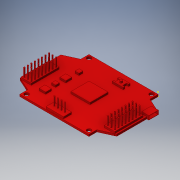
# Autodesk Inventor part: control board
Saved by Autodesk Inventor 2016 (Build 200138000, 138)
## iProperties
Created: 2015-05-25
Part Number: control board
Material: Generic
Document SubType Name: Modeling
Designer: Admin
Density: 1 g/cm^3
Appearance: Default
Mass: 5.47017 g
Surface Area: 80.281 cm^2
Volume: 5.47017 cm^3
Author: Admin
Autodesk Inventor part; units mm, degrees
ref_plane "YZ Plane" through (0, 0, 0) normal (1, 0, 0) x (0, 1, 0)
ref_plane "XZ Plane" through (0, 0, 0) normal (0, 1, 0) x (-1, 0, 0)
ref_plane "XY Plane" through (0, 0, 0) normal (0, 0, 1) x (1, 0, 0)
sketch "Sketch1" plane through (0, 0, 0) normal (0, 1, 0) x (-1, 0, 0)
  circle A0 centre (2.3047, 47.3782) radius 1.524
  line L0 (-0.1112, 0.0907) -> (-0.1112, 49.8747)
  line L1 (-0.1112, 49.8747) -> (-0.1112, 44.1597)
  line L2 (-0.1112, 44.1597) -> (-9.996, 39.6997)
  line L3 (-9.996, 10.5342) -> (-0.1112, 6.0187)
  circle A1 centre (47.3135, 47.3513) radius 1.524
  line L4 (49.6728, 0.0907) -> (49.7323, 49.845)
  line L5 (49.7323, 49.845) -> (49.7255, 44.1597)
  line L6 (49.7255, 44.1597) -> (59.6049, 39.6878)
  line L7 (59.6049, 39.6878) -> (59.5701, 10.5224)
  line L8 (59.5701, 10.5224) -> (49.6799, 6.0187)
  circle A2 centre (21.0522, 45.994) radius 0.4445
  circle A3 centre (23.6023, 45.9907) radius 0.4445
  circle A4 centre (26.1324, 46.0137) radius 0.4445
  circle A5 centre (28.6839, 46.0031) radius 0.4445
  line L9 (-1.4472, 40.2524) -> (-9.0679, 40.2524)
  line L10 (-9.0679, 40.2524) -> (-9.0679, 19.9143)
  line L11 (-9.0679, 19.9143) -> (-1.4472, 19.9143)
  line L12 (-1.4472, 19.9143) -> (-1.4472, 40.2524)
  line L13 (51.1741, 40.1712) -> (58.7055, 40.1712)
  line L14 (58.7055, 40.1712) -> (58.7055, 20.0074)
  line L15 (58.7055, 20.0074) -> (51.1741, 20.0074)
  line L16 (51.1741, 20.0074) -> (51.1741, 40.1712)
  line L17 (18.5986, 43.6399) -> (31.2098, 43.6399)
  line L18 (31.2098, 43.6399) -> (31.2098, 49.4826)
  line L19 (31.2098, 49.4826) -> (18.5986, 49.4901)
  line L20 (18.5986, 49.4901) -> (18.5986, 43.6399)
  line L21 (17.9249, 31.092) -> (31.6611, 31.092)
  line L22 (31.6611, 31.092) -> (31.6611, 18.0268)
  line L23 (31.6611, 18.0268) -> (17.9249, 18.0268)
  line L24 (17.9249, 18.0268) -> (17.9249, 31.092)
  circle A6 centre (-5.2821, 38.9142) radius 0.4445
  circle A7 centre (-2.7297, 38.9142) radius 0.4445
  circle A8 centre (-7.7994, 38.9142) radius 0.4445
  circle A9 centre (-5.2821, 36.3742) radius 0.4445
  circle A10 centre (-2.7297, 36.3742) radius 0.4445
  circle A11 centre (-7.7994, 36.3742) radius 0.4445
  circle A12 centre (-5.2821, 33.8342) radius 0.4445
  circle A13 centre (-2.7297, 33.8342) radius 0.4445
  circle A14 centre (-7.7994, 33.8342) radius 0.4445
  circle A15 centre (-5.2821, 31.2942) radius 0.4445
  circle A16 centre (-2.7297, 31.2942) radius 0.4445
  circle A17 centre (-7.7994, 31.2942) radius 0.4445
  circle A18 centre (-5.2821, 21.1342) radius 0.4445
  circle A19 centre (-2.7297, 21.1342) radius 0.4445
  circle A20 centre (-7.7994, 21.1342) radius 0.4445
  circle A21 centre (-5.2821, 23.6742) radius 0.4445
  circle A22 centre (-2.7297, 23.6742) radius 0.4445
  circle A23 centre (-7.7994, 23.6742) radius 0.4445
  circle A24 centre (-5.2821, 26.2142) radius 0.4445
  circle A25 centre (-2.7297, 26.2142) radius 0.4445
  circle A26 centre (-7.7994, 26.2142) radius 0.4445
  circle A27 centre (-5.2821, 28.7542) radius 0.4445
  circle A28 centre (-2.7297, 28.7542) radius 0.4445
  circle A29 centre (-7.7994, 28.7542) radius 0.4445
  circle A30 centre (54.8719, 38.9142) radius 0.4445
  circle A31 centre (52.3196, 38.9142) radius 0.4445
  circle A32 centre (57.3893, 38.9142) radius 0.4445
  circle A33 centre (54.8719, 36.3742) radius 0.4445
  circle A34 centre (52.3196, 36.3742) radius 0.4445
  circle A35 centre (57.3893, 36.3742) radius 0.4445
  circle A36 centre (54.8719, 33.8342) radius 0.4445
  circle A37 centre (52.3196, 33.8342) radius 0.4445
  circle A38 centre (57.3893, 33.8342) radius 0.4445
  circle A39 centre (54.8719, 31.2942) radius 0.4445
  circle A40 centre (52.3196, 31.2942) radius 0.4445
  circle A41 centre (57.3893, 31.2942) radius 0.4445
  circle A42 centre (54.8719, 21.1342) radius 0.4445
  circle A43 centre (52.3196, 21.1342) radius 0.4445
  circle A44 centre (57.3893, 21.1342) radius 0.4445
  circle A45 centre (54.8719, 23.6742) radius 0.4445
  circle A46 centre (52.3196, 23.6742) radius 0.4445
  circle A47 centre (57.3893, 23.6742) radius 0.4445
  circle A48 centre (54.8719, 26.2142) radius 0.4445
  circle A49 centre (52.3196, 26.2142) radius 0.4445
  circle A50 centre (57.3893, 26.2142) radius 0.4445
  circle A51 centre (54.8719, 28.7542) radius 0.4445
  circle A52 centre (52.3196, 28.7542) radius 0.4445
  circle A53 centre (57.3893, 28.7542) radius 0.4445
  line L25 (15.3968, 9.7927) -> (23.2335, 9.7927)
  line L26 (23.2335, 9.7927) -> (23.2335, 8.6499)
  line L27 (23.2335, 8.6499) -> (21.8717, 8.6499)
  line L28 (21.8717, 8.6499) -> (21.8717, 5.9895)
  line L29 (21.8717, 5.9895) -> (23.2215, 5.9895)
  line L30 (23.2215, 5.9895) -> (23.2215, 4.7481)
  line L31 (23.2215, 4.7481) -> (15.3804, 4.7481)
  line L32 (15.3804, 4.7481) -> (15.3804, 5.8201)
  line L33 (15.3804, 5.8201) -> (16.855, 5.8201)
  line L34 (16.855, 5.8201) -> (16.855, 8.6339)
  line L35 (16.855, 8.6339) -> (15.3133, 8.6339)
  line L36 (15.3133, 8.6339) -> (15.3133, 9.7894)
  line L37 (15.3968, 9.7927) -> (15.3133, 9.7927)
  line L38 (15.3133, 9.7894) -> (15.3133, 9.7927)
  circle A54 centre (19.4197, 7.2385) radius 0.9144
  line L39 (40.3965, 40.5916) -> (45.1465, 40.5916)
  line L40 (45.1465, 40.5916) -> (45.1465, 36.3389)
  line L41 (45.1465, 36.3389) -> (40.3965, 36.3389)
  line L42 (40.3965, 36.3389) -> (40.3965, 40.5916)
  line L43 (41.1619, 32.6713) -> (44.0659, 32.6713)
  line L44 (44.0659, 32.6713) -> (44.0659, 29.7688)
  line L45 (44.0659, 29.7688) -> (41.1619, 29.7688)
  line L46 (41.1619, 29.7688) -> (41.1619, 32.6713)
  line L47 (40.2197, 26.2622) -> (44.5432, 26.2622)
  line L48 (44.5432, 26.2622) -> (44.5432, 21.9124)
  line L49 (44.5432, 21.9124) -> (40.2197, 21.9124)
  line L50 (40.2197, 21.9124) -> (40.2197, 26.2622)
  line L51 (40.1066, 16.8549) -> (42.9715, 16.8549)
  line L52 (42.9715, 16.8549) -> (42.9715, 13.9684)
  line L53 (42.9715, 13.9684) -> (40.1066, 13.9684)
  line L54 (40.1066, 13.9684) -> (40.1066, 16.8549)
  circle A55 centre (2.3047, 2.3694) radius 1.524
  circle A56 centre (47.3135, 2.3694) radius 1.524
  line L55 (-6.3047, 18.0939) -> (-11.4234, 18.0939)
  line L56 (-11.4234, 18.0939) -> (-11.4234, 11.2092)
  line L57 (-11.4234, 11.2092) -> (-6.3047, 11.2092)
  line L58 (-6.3047, 11.2092) -> (-6.3047, 18.0939)
  line L59 (-9.996, 39.6997) -> (-9.996, 18.0939)
  line L60 (-9.996, 11.2092) -> (-9.996, 10.5342)
  line L61 (49.7323, 49.845) -> (-0.1112, 49.8747)
  line L62 (-0.1112, 0.0907) -> (49.6728, 0.0907)
  constraints: 126 end point, 57 centre point, 54 equal radius, 6 point on line, 3 parallel, 1 horizontal
extrude "Extrusion1" add sketch "Sketch1" along normal blind 1.4 contours L0 L61 L4 L62 | L3 L60 L57 L58 L55 L59 L2 L10 L11 L12 L9 L0 | L4 L6 L13 L16 L15 L14 L7 L8 | L9 L12 L11 L10 L2 | L6 L14 L15 L16 L13
sketch "Sketch2" plane through (0, 0, 0) normal (0, 1, 0) x (-1, 0, 0)
  circle A0 centre (2.3047, 47.3782) radius 1.524
  line L0 (-0.1112, 0.0907) -> (-0.1112, 49.8747)
  line L1 (-0.1112, 49.8747) -> (-0.1112, 44.1597)
  line L2 (-0.1112, 44.1597) -> (-9.996, 39.6997)
  line L3 (-9.996, 10.5342) -> (-0.1112, 6.0187)
  circle A1 centre (47.3135, 47.3513) radius 1.524
  line L4 (49.6728, 0.0907) -> (49.7323, 49.845)
  line L5 (49.7323, 49.845) -> (49.7255, 44.1597)
  line L6 (49.7255, 44.1597) -> (59.6049, 39.6878)
  line L7 (59.6049, 39.6878) -> (59.5701, 10.5224)
  line L8 (59.5701, 10.5224) -> (49.6799, 6.0187)
  circle A2 centre (21.0522, 45.994) radius 0.4445
  circle A3 centre (23.6023, 45.9907) radius 0.4445
  circle A4 centre (26.1324, 46.0137) radius 0.4445
  circle A5 centre (28.6839, 46.0031) radius 0.4445
  line L9 (-1.4472, 40.2524) -> (-9.0679, 40.2524)
  line L10 (-9.0679, 40.2524) -> (-9.0679, 19.9143)
  line L11 (-9.0679, 19.9143) -> (-1.4472, 19.9143)
  line L12 (-1.4472, 19.9143) -> (-1.4472, 40.2524)
  line L13 (51.1741, 40.1712) -> (58.7055, 40.1712)
  line L14 (58.7055, 40.1712) -> (58.7055, 20.0074)
  line L15 (58.7055, 20.0074) -> (51.1741, 20.0074)
  line L16 (51.1741, 20.0074) -> (51.1741, 40.1712)
  line L17 (18.5986, 43.6399) -> (31.2098, 43.6399)
  line L18 (31.2098, 43.6399) -> (31.2098, 49.4826)
  line L19 (31.2098, 49.4826) -> (18.5986, 49.4901)
  line L20 (18.5986, 49.4901) -> (18.5986, 43.6399)
  line L21 (17.9249, 31.092) -> (31.6611, 31.092)
  line L22 (31.6611, 31.092) -> (31.6611, 18.0268)
  line L23 (31.6611, 18.0268) -> (17.9249, 18.0268)
  line L24 (17.9249, 18.0268) -> (17.9249, 31.092)
  circle A6 centre (-5.2821, 38.9142) radius 0.4445
  circle A7 centre (-2.7297, 38.9142) radius 0.4445
  circle A8 centre (-7.7994, 38.9142) radius 0.4445
  circle A9 centre (-5.2821, 36.3742) radius 0.4445
  circle A10 centre (-2.7297, 36.3742) radius 0.4445
  circle A11 centre (-7.7994, 36.3742) radius 0.4445
  circle A12 centre (-5.2821, 33.8342) radius 0.4445
  circle A13 centre (-2.7297, 33.8342) radius 0.4445
  circle A14 centre (-7.7994, 33.8342) radius 0.4445
  circle A15 centre (-5.2821, 31.2942) radius 0.4445
  circle A16 centre (-2.7297, 31.2942) radius 0.4445
  circle A17 centre (-7.7994, 31.2942) radius 0.4445
  circle A18 centre (-5.2821, 21.1342) radius 0.4445
  circle A19 centre (-2.7297, 21.1342) radius 0.4445
  circle A20 centre (-7.7994, 21.1342) radius 0.4445
  circle A21 centre (-5.2821, 23.6742) radius 0.4445
  circle A22 centre (-2.7297, 23.6742) radius 0.4445
  circle A23 centre (-7.7994, 23.6742) radius 0.4445
  circle A24 centre (-5.2821, 26.2142) radius 0.4445
  circle A25 centre (-2.7297, 26.2142) radius 0.4445
  circle A26 centre (-7.7994, 26.2142) radius 0.4445
  circle A27 centre (-5.2821, 28.7542) radius 0.4445
  circle A28 centre (-2.7297, 28.7542) radius 0.4445
  circle A29 centre (-7.7994, 28.7542) radius 0.4445
  circle A30 centre (54.8719, 38.9142) radius 0.4445
  circle A31 centre (52.3196, 38.9142) radius 0.4445
  circle A32 centre (57.3893, 38.9142) radius 0.4445
  circle A33 centre (54.8719, 36.3742) radius 0.4445
  circle A34 centre (52.3196, 36.3742) radius 0.4445
  circle A35 centre (57.3893, 36.3742) radius 0.4445
  circle A36 centre (54.8719, 33.8342) radius 0.4445
  circle A37 centre (52.3196, 33.8342) radius 0.4445
  circle A38 centre (57.3893, 33.8342) radius 0.4445
  circle A39 centre (54.8719, 31.2942) radius 0.4445
  circle A40 centre (52.3196, 31.2942) radius 0.4445
  circle A41 centre (57.3893, 31.2942) radius 0.4445
  circle A42 centre (54.8719, 21.1342) radius 0.4445
  circle A43 centre (52.3196, 21.1342) radius 0.4445
  circle A44 centre (57.3893, 21.1342) radius 0.4445
  circle A45 centre (54.8719, 23.6742) radius 0.4445
  circle A46 centre (52.3196, 23.6742) radius 0.4445
  circle A47 centre (57.3893, 23.6742) radius 0.4445
  circle A48 centre (54.8719, 26.2142) radius 0.4445
  circle A49 centre (52.3196, 26.2142) radius 0.4445
  circle A50 centre (57.3893, 26.2142) radius 0.4445
  circle A51 centre (54.8719, 28.7542) radius 0.4445
  circle A52 centre (52.3196, 28.7542) radius 0.4445
  circle A53 centre (57.3893, 28.7542) radius 0.4445
  line L25 (15.3968, 9.7927) -> (23.2335, 9.7927)
  line L26 (23.2335, 9.7927) -> (23.2335, 8.6499)
  line L27 (23.2335, 8.6499) -> (21.8717, 8.6499)
  line L28 (21.8717, 8.6499) -> (21.8717, 5.9895)
  line L29 (21.8717, 5.9895) -> (23.2215, 5.9895)
  line L30 (23.2215, 5.9895) -> (23.2215, 4.7481)
  line L31 (23.2215, 4.7481) -> (15.3804, 4.7481)
  line L32 (15.3804, 4.7481) -> (15.3804, 5.8201)
  line L33 (15.3804, 5.8201) -> (16.855, 5.8201)
  line L34 (16.855, 5.8201) -> (16.855, 8.6339)
  line L35 (16.855, 8.6339) -> (15.3133, 8.6339)
  line L36 (15.3133, 8.6339) -> (15.3133, 9.7894)
  line L37 (15.3968, 9.7927) -> (15.3133, 9.7927)
  line L38 (15.3133, 9.7894) -> (15.3133, 9.7927)
  circle A54 centre (19.4197, 7.2385) radius 0.9144
  line L39 (40.3965, 40.5916) -> (45.1465, 40.5916)
  line L40 (45.1465, 40.5916) -> (45.1465, 36.3389)
  line L41 (45.1465, 36.3389) -> (40.3965, 36.3389)
  line L42 (40.3965, 36.3389) -> (40.3965, 40.5916)
  line L43 (41.1619, 32.6713) -> (44.0659, 32.6713)
  line L44 (44.0659, 32.6713) -> (44.0659, 29.7688)
  line L45 (44.0659, 29.7688) -> (41.1619, 29.7688)
  line L46 (41.1619, 29.7688) -> (41.1619, 32.6713)
  line L47 (40.2197, 26.2622) -> (44.5432, 26.2622)
  line L48 (44.5432, 26.2622) -> (44.5432, 21.9124)
  line L49 (44.5432, 21.9124) -> (40.2197, 21.9124)
  line L50 (40.2197, 21.9124) -> (40.2197, 26.2622)
  line L51 (40.1066, 16.8549) -> (42.9715, 16.8549)
  line L52 (42.9715, 16.8549) -> (42.9715, 13.9684)
  line L53 (42.9715, 13.9684) -> (40.1066, 13.9684)
  line L54 (40.1066, 13.9684) -> (40.1066, 16.8549)
  circle A55 centre (2.3047, 2.3694) radius 1.524
  circle A56 centre (47.3135, 2.3694) radius 1.524
  line L55 (-6.3047, 18.0939) -> (-11.4234, 18.0939)
  line L56 (-11.4234, 18.0939) -> (-11.4234, 11.2092)
  line L57 (-11.4234, 11.2092) -> (-6.3047, 11.2092)
  line L58 (-6.3047, 11.2092) -> (-6.3047, 18.0939)
  line L59 (-9.996, 39.6997) -> (-9.996, 18.0939)
  line L60 (-9.996, 11.2092) -> (-9.996, 10.5342)
  line L61 (49.7323, 49.845) -> (-0.1112, 49.8747)
  line L62 (-0.1112, 0.0907) -> (49.6728, 0.0907)
  point P0 (0, 0)
  constraints: 126 end point, 57 centre point, 54 equal radius, 6 point on line, 3 parallel, 1 horizontal
extrude "Extrusion2" add sketch "Sketch2" along normal blind 2.8 contours L9 L12 L11 L10 L2 | L2 L10 L9 | L57 L56 L55 L58 | L13 L14 L6 | L6 L14 L15 L16 L13 | L20 L19 L18 L17 | L21 L22 L23 L24 | L25 L26 L27 L28 L29 L30 L31 L32 L33 L34 L35 L36 L38 L37 | L39 L40 L41 L42 | L43 L44 L45 L46 | L47 L48 L49 L50 | L51 L52 L53 L54
sketch "Sketch3" plane through (0, 0, 0) normal (0, 0, 1) x (1, 0, 0)
  point P0 (0, 0)
sketch "Sketch4" plane through (0, 0, 0) normal (0, 1, 0) x (-1, 0, 0)
  circle A0 centre (2.3047, 47.3782) radius 1.524
  line L0 (-0.1112, 0.0907) -> (-0.1112, 49.8747)
  line L1 (-0.1112, 49.8747) -> (-0.1112, 44.1597)
  line L2 (-0.1112, 44.1597) -> (-9.996, 39.6997)
  line L3 (-9.996, 10.5342) -> (-0.1112, 6.0187)
  circle A1 centre (47.3135, 47.3513) radius 1.524
  line L4 (49.6728, 0.0907) -> (49.7323, 49.845)
  line L5 (49.7323, 49.845) -> (49.7255, 44.1597)
  line L6 (49.7255, 44.1597) -> (59.6049, 39.6878)
  line L7 (59.6049, 39.6878) -> (59.5701, 10.5224)
  line L8 (59.5701, 10.5224) -> (49.6799, 6.0187)
  circle A2 centre (21.0522, 45.994) radius 0.4445
  circle A3 centre (23.6023, 45.9907) radius 0.4445
  circle A4 centre (26.1324, 46.0137) radius 0.4445
  circle A5 centre (28.6839, 46.0031) radius 0.4445
  line L9 (-1.4472, 40.2524) -> (-9.0679, 40.2524)
  line L10 (-9.0679, 40.2524) -> (-9.0679, 19.9143)
  line L11 (-9.0679, 19.9143) -> (-1.4472, 19.9143)
  line L12 (-1.4472, 19.9143) -> (-1.4472, 40.2524)
  line L13 (51.1741, 40.1712) -> (58.7055, 40.1712)
  line L14 (58.7055, 40.1712) -> (58.7055, 20.0074)
  line L15 (58.7055, 20.0074) -> (51.1741, 20.0074)
  line L16 (51.1741, 20.0074) -> (51.1741, 40.1712)
  line L17 (18.5986, 43.6399) -> (31.2098, 43.6399)
  line L18 (31.2098, 43.6399) -> (31.2098, 49.4826)
  line L19 (31.2098, 49.4826) -> (18.5986, 49.4901)
  line L20 (18.5986, 49.4901) -> (18.5986, 43.6399)
  line L21 (17.9249, 31.092) -> (31.6611, 31.092)
  line L22 (31.6611, 31.092) -> (31.6611, 18.0268)
  line L23 (31.6611, 18.0268) -> (17.9249, 18.0268)
  line L24 (17.9249, 18.0268) -> (17.9249, 31.092)
  circle A6 centre (-5.2821, 38.9142) radius 0.4445
  circle A7 centre (-2.7297, 38.9142) radius 0.4445
  circle A8 centre (-7.7994, 38.9142) radius 0.4445
  circle A9 centre (-5.2821, 36.3742) radius 0.4445
  circle A10 centre (-2.7297, 36.3742) radius 0.4445
  circle A11 centre (-7.7994, 36.3742) radius 0.4445
  circle A12 centre (-5.2821, 33.8342) radius 0.4445
  circle A13 centre (-2.7297, 33.8342) radius 0.4445
  circle A14 centre (-7.7994, 33.8342) radius 0.4445
  circle A15 centre (-5.2821, 31.2942) radius 0.4445
  circle A16 centre (-2.7297, 31.2942) radius 0.4445
  circle A17 centre (-7.7994, 31.2942) radius 0.4445
  circle A18 centre (-5.2821, 21.1342) radius 0.4445
  circle A19 centre (-2.7297, 21.1342) radius 0.4445
  circle A20 centre (-7.7994, 21.1342) radius 0.4445
  circle A21 centre (-5.2821, 23.6742) radius 0.4445
  circle A22 centre (-2.7297, 23.6742) radius 0.4445
  circle A23 centre (-7.7994, 23.6742) radius 0.4445
  circle A24 centre (-5.2821, 26.2142) radius 0.4445
  circle A25 centre (-2.7297, 26.2142) radius 0.4445
  circle A26 centre (-7.7994, 26.2142) radius 0.4445
  circle A27 centre (-5.2821, 28.7542) radius 0.4445
  circle A28 centre (-2.7297, 28.7542) radius 0.4445
  circle A29 centre (-7.7994, 28.7542) radius 0.4445
  circle A30 centre (54.8719, 38.9142) radius 0.4445
  circle A31 centre (52.3196, 38.9142) radius 0.4445
  circle A32 centre (57.3893, 38.9142) radius 0.4445
  circle A33 centre (54.8719, 36.3742) radius 0.4445
  circle A34 centre (52.3196, 36.3742) radius 0.4445
  circle A35 centre (57.3893, 36.3742) radius 0.4445
  circle A36 centre (54.8719, 33.8342) radius 0.4445
  circle A37 centre (52.3196, 33.8342) radius 0.4445
  circle A38 centre (57.3893, 33.8342) radius 0.4445
  circle A39 centre (54.8719, 31.2942) radius 0.4445
  circle A40 centre (52.3196, 31.2942) radius 0.4445
  circle A41 centre (57.3893, 31.2942) radius 0.4445
  circle A42 centre (54.8719, 21.1342) radius 0.4445
  circle A43 centre (52.3196, 21.1342) radius 0.4445
  circle A44 centre (57.3893, 21.1342) radius 0.4445
  circle A45 centre (54.8719, 23.6742) radius 0.4445
  circle A46 centre (52.3196, 23.6742) radius 0.4445
  circle A47 centre (57.3893, 23.6742) radius 0.4445
  circle A48 centre (54.8719, 26.2142) radius 0.4445
  circle A49 centre (52.3196, 26.2142) radius 0.4445
  circle A50 centre (57.3893, 26.2142) radius 0.4445
  circle A51 centre (54.8719, 28.7542) radius 0.4445
  circle A52 centre (52.3196, 28.7542) radius 0.4445
  circle A53 centre (57.3893, 28.7542) radius 0.4445
  line L25 (15.3968, 9.7927) -> (23.2335, 9.7927)
  line L26 (23.2335, 9.7927) -> (23.2335, 8.6499)
  line L27 (23.2335, 8.6499) -> (21.8717, 8.6499)
  line L28 (21.8717, 8.6499) -> (21.8717, 5.9895)
  line L29 (21.8717, 5.9895) -> (23.2215, 5.9895)
  line L30 (23.2215, 5.9895) -> (23.2215, 4.7481)
  line L31 (23.2215, 4.7481) -> (15.3804, 4.7481)
  line L32 (15.3804, 4.7481) -> (15.3804, 5.8201)
  line L33 (15.3804, 5.8201) -> (16.855, 5.8201)
  line L34 (16.855, 5.8201) -> (16.855, 8.6339)
  line L35 (16.855, 8.6339) -> (15.3133, 8.6339)
  line L36 (15.3133, 8.6339) -> (15.3133, 9.7894)
  line L37 (15.3968, 9.7927) -> (15.3133, 9.7927)
  line L38 (15.3133, 9.7894) -> (15.3133, 9.7927)
  circle A54 centre (19.4197, 7.2385) radius 0.9144
  line L39 (40.3965, 40.5916) -> (45.1465, 40.5916)
  line L40 (45.1465, 40.5916) -> (45.1465, 36.3389)
  line L41 (45.1465, 36.3389) -> (40.3965, 36.3389)
  line L42 (40.3965, 36.3389) -> (40.3965, 40.5916)
  line L43 (41.1619, 32.6713) -> (44.0659, 32.6713)
  line L44 (44.0659, 32.6713) -> (44.0659, 29.7688)
  line L45 (44.0659, 29.7688) -> (41.1619, 29.7688)
  line L46 (41.1619, 29.7688) -> (41.1619, 32.6713)
  line L47 (40.2197, 26.2622) -> (44.5432, 26.2622)
  line L48 (44.5432, 26.2622) -> (44.5432, 21.9124)
  line L49 (44.5432, 21.9124) -> (40.2197, 21.9124)
  line L50 (40.2197, 21.9124) -> (40.2197, 26.2622)
  line L51 (40.1066, 16.8549) -> (42.9715, 16.8549)
  line L52 (42.9715, 16.8549) -> (42.9715, 13.9684)
  line L53 (42.9715, 13.9684) -> (40.1066, 13.9684)
  line L54 (40.1066, 13.9684) -> (40.1066, 16.8549)
  circle A55 centre (2.3047, 2.3694) radius 1.524
  circle A56 centre (47.3135, 2.3694) radius 1.524
  line L55 (-6.3047, 18.0939) -> (-11.4234, 18.0939)
  line L56 (-11.4234, 18.0939) -> (-11.4234, 11.2092)
  line L57 (-11.4234, 11.2092) -> (-6.3047, 11.2092)
  line L58 (-6.3047, 11.2092) -> (-6.3047, 18.0939)
  line L59 (-9.996, 39.6997) -> (-9.996, 18.0939)
  line L60 (-9.996, 11.2092) -> (-9.996, 10.5342)
  line L61 (49.7323, 49.845) -> (-0.1112, 49.8747)
  line L62 (-0.1112, 0.0907) -> (49.6728, 0.0907)
  point P0 (0, 0)
  constraints: 126 end point, 57 centre point, 54 equal radius, 6 point on line, 3 parallel, 1 horizontal
extrude "Extrusion3" add sketch "Sketch4" along normal blind 8.89 contours A2 | A3 | A4 | A5 | A6 | A7 | A8 | A9 | A10 | A11 | A12 | A13 | A14 | A15 | A16 | A17 | A18 | A19 | A20 | A21 | A22 | A23 | A24 | A25 | A26 | A27 | A28 | A29 | A30 | A31 | A32 | A33 | A34 | A35 | A36 | A37 | A38 | A39 | A40 | A41 | A42 | A43 | A44 | A45 | A46 | A47 | A48 | A49 | A50 | A51 | A52 | A53
sketch "Sketch5" plane through (11.4234, 0, 18.0939) normal (1, 0, 0) x (0, 0, -1)
  line L0 (0.0671, 1.4) -> (0.0671, 2.8) projected
  line L1 (7.5715, 0) -> (-21.5939, 0) projected
  line L2 (0.0671, 2.8) -> (6.9117, 2.8)
  line L3 (6.9117, 2.8) -> (6.9117, 0)
  line L4 (6.9117, 0) -> (0.0671, 0)
  line L5 (0.0671, 0) -> (0.0671, 2.8)
  line L6 (0.254, 0.2397) -> (6.7248, 0.2397)
  line L7 (6.7248, 0.2397) -> (6.7248, 2.5603)
  line L8 (6.7248, 2.5603) -> (0.254, 2.5603)
  line L9 (0.254, 2.5603) -> (0.254, 0.2397)
  line L10 (7.5715, 1.4) -> (-21.5939, 1.4) projected
  line L11 (0.254, 0.2397) -> (6.7248, 2.5603) construction
  line L12 (6.7248, 0.2397) -> (0.254, 2.5603) construction
  point P0 (18.0939, 0)
  point P1 (3.4894, 1.4)
  constraints: 20 end point, 4 parallel, 2 horizontal, 2 midpoint, 2 perpendicular, 2 point on line
sketch "Sketch6" plane through (0, 2.8, 0) normal (0, 1, 0) x (1, 0, 0)
  point P0 (0, 0)
extrude "Extrusion4" cut sketch "Sketch5" against normal blind 4.064 contours L10 L7 L6 L9 | L9 L8 L7 L10
sketch "Sketch7" plane through (0, 2.8, 0) normal (0, 1, 0) x (1, 0, 0)
  circle A0 centre (-19.4197, -7.2385) radius 0.9144 projected
  circle A1 centre (-19.4197, -7.2385) radius 0.9144
  point P0 (0, 0)
  constraints: 1 centre point, 1 coincident
extrude "Extrusion5" add sketch "Sketch7" along normal mid plane 2.54
sketch "Sketch8" plane through (0, 0, 0) normal (0, -1, 0) x (1, 0, 0)
  point P0 (0, 0)
sketch "Sketch9" plane through (-19.4197, 1.53, 7.2385) normal (0, -1, 0) x (1, 0, 0)
  circle A0 centre (0, 0) radius 0.9144 projected
  circle A1 centre (0, 0) radius 0.9144
  point P0 (19.4197, -7.2385)
  constraints: 1 centre point, 1 coincident
extrude "Extrusion6" add sketch "Sketch9" along normal blind 1.53
sketch "Sketch10" plane through (-26.1324, 8.89, 46.0137) normal (0, 1, 0) x (1, 0, 0)
  point P0 (26.1324, 46.0137)
body "Solid1"
